Autodesk Fusion 360 part; units mm, degrees
(part 2 of 2)
sketch "Sketch5" plane through (0, 0, 0) normal (0, 0, 1) x (1, 0, 0)
  circle A0 centre (0, 0) radius 99.7546
  line L0 (-24.2133, 222.1165) -> (-40.213, 240.9922)
  arc A1 (-40.213, 240.9922) -> (-47.0298, 239.7551) centre (-43.2643, 238.4058) ccw
  line L1 (-47.0298, 239.7551) -> (-55.3768, 216.4612)
  arc A2 (-58.0942, 213.9503) -> (-55.3768, 216.4612) centre (-59.1424, 217.8105) ccw
  arc A3 (-58.0942, 213.9503) -> (-59.8641, 213.4618) centre (0, 0) ccw
  arc A4 (-63.4846, 214.2236) -> (-59.8641, 213.4618) centre (-60.9442, 217.3132) ccw
  line L2 (-63.4846, 214.2236) -> (-82.5975, 229.9391)
  arc A5 (-82.5975, 229.9391) -> (-89.084, 227.5047) centre (-85.138, 226.8494) ccw
  line L3 (-89.084, 227.5047) -> (-93.1375, 203.0946)
  arc A6 (-95.3629, 200.1389) -> (-93.1375, 203.0946) centre (-97.0835, 203.7499) ccw
  arc A7 (-95.3629, 200.1389) -> (-97.0171, 199.3423) centre (0, 0) ccw
  arc A8 (-100.7155, 199.4453) -> (-97.0171, 199.3423) centre (-98.7675, 202.9389) ccw
  line L4 (-100.7155, 199.4453) -> (-122.3274, 211.4955)
  arc A9 (-122.3274, 211.4955) -> (-128.2749, 207.942) centre (-124.2753, 208.0019) ccw
  line L5 (-128.2749, 207.942) -> (-127.9047, 183.2005)
  arc A10 (-129.5665, 179.8949) -> (-127.9047, 183.2005) centre (-131.9043, 183.1406) ccw
  arc A11 (-129.5665, 179.8949) -> (-131.0519, 178.8157) centre (0, 0) ccw
  arc A12 (-134.7093, 178.2567) -> (-131.0519, 178.8157) centre (-133.4164, 182.042) ccw
  line L6 (-134.7093, 178.2567) -> (-158.1255, 186.2543)
  arc A13 (-158.1255, 186.2543) -> (-163.3429, 181.6959) centre (-159.4183, 182.469) ccw
  line L7 (-163.3429, 181.6959) -> (-158.5609, 157.4181)
  arc A14 (-159.6058, 153.8689) -> (-158.5609, 157.4181) centre (-162.4855, 156.6451) ccw
  arc A15 (-159.6058, 153.8689) -> (-160.8746, 152.5418) centre (0, 0) ccw
  arc A16 (-164.3734, 151.3387) -> (-160.8746, 152.5418) centre (-163.7772, 155.2941) ccw
  line L8 (-164.3734, 151.3387) -> (-188.8413, 155.0267)
  arc A17 (-188.8413, 155.0267) -> (-193.161, 149.61) centre (-189.4375, 151.0714) ccw
  line L9 (-193.161, 149.61) -> (-184.1209, 126.5762)
  arc A18 (-184.5152, 122.8974) -> (-184.1209, 126.5762) centre (-187.8444, 125.1148) ccw
  arc A19 (-184.5152, 122.8974) -> (-185.5267, 121.3651) centre (0, 0) ccw
  arc A20 (-188.7544, 119.5567) -> (-185.5267, 121.3651) centre (-188.8741, 123.5549) ccw
  line L10 (-188.7544, 119.5567) -> (-213.4877, 118.8164)
  arc A21 (-213.4877, 118.8164) -> (-216.7707, 112.7155) centre (-213.368, 114.8182) ccw
  line L11 (-216.7707, 112.7155) -> (-203.763, 91.666)
  arc A22 (-203.4942, 87.9759) -> (-203.763, 91.666) centre (-207.1658, 89.5633) ccw
  arc A23 (-203.4942, 87.9759) -> (-204.2158, 86.2877) centre (0, 0) ccw
  arc A24 (-207.0687, 83.9319) -> (-204.2158, 86.2877) centre (-207.9004, 87.8445) ccw
  line L12 (-207.0687, 83.9319) -> (-231.2723, 78.7873)
  arc A25 (-231.2723, 78.7873) -> (-233.4133, 72.1982) centre (-230.4407, 74.8747) ccw
  line L13 (-233.4133, 72.1982) -> (-216.8561, 53.8096)
  arc A26 (-215.9327, 50.2268) -> (-216.8561, 53.8096) centre (-219.8287, 51.1331) ccw
  arc A27 (-215.9327, 50.2268) -> (-216.3412, 48.4369) centre (0, 0) ccw
  arc A28 (-218.7277, 45.6096) -> (-216.3412, 48.4369) centre (-220.2446, 49.3108) ccw
  line L14 (-218.7277, 45.6096) -> (-241.6237, 36.2259)
  arc A29 (-241.6237, 36.2259) -> (-242.5537, 29.3604) centre (-240.1068, 32.5247) ccw
  line L15 (-242.5537, 29.3604) -> (-222.9792, 14.2237)
  arc A30 (-221.4309, 10.8634) -> (-222.9792, 14.2237) centre (-225.4261, 11.0594) ccw
  arc A31 (-221.4309, 10.8634) -> (-221.5133, 9.0292) centre (0, 0) ccw
  arc A32 (-223.3565, 5.8213) -> (-221.5133, 9.0292) centre (-225.51, 9.1921) ccw
  line L16 (-223.3565, 5.8213) -> (-244.2091, -7.4998)
  arc A33 (-244.2091, -7.4998) -> (-243.8983, -14.4211) centre (-242.0557, -10.8707) ccw
  line L17 (-243.8983, -14.4211) -> (-221.9356, -25.8194)
  arc A34 (-219.8121, -28.8492) -> (-221.9356, -25.8194) centre (-223.7781, -29.3697) ccw
  arc A35 (-219.8121, -28.8492) -> (-219.5657, -30.6686) centre (0, 0) ccw
  arc A36 (-220.8065, -34.1541) -> (-219.5657, -30.6686) centre (-223.5272, -31.2219) ccw
  line L18 (-220.8065, -34.1541) -> (-238.9454, -50.9845)
  arc A37 (-238.9454, -50.9845) -> (-237.4037, -57.739) centre (-236.2247, -53.9167) ccw
  line L19 (-237.4037, -57.739) -> (-213.7587, -65.0326)
  arc A38 (-211.1285, -67.6345) -> (-213.7587, -65.0326) centre (-214.9378, -68.8548) ccw
  arc A39 (-211.1285, -67.6345) -> (-210.5611, -69.3807) centre (0, 0) ccw
  arc A40 (-211.1596, -73.0318) -> (-210.5611, -69.3807) centre (-214.3602, -70.6325) ccw
  line L20 (-211.1596, -73.0318) -> (-226.0018, -92.8305)
  arc A41 (-226.0018, -92.8305) -> (-223.2788, -99.2012) centre (-222.8013, -95.2298) ccw
  line L21 (-223.2788, -99.2012) -> (-198.7115, -102.1555)
  arc A42 (-195.6589, -104.2461) -> (-198.7115, -102.1555) centre (-199.1891, -106.1269) ccw
  arc A43 (-195.6589, -104.2461) -> (-194.7889, -105.8629) centre (0, 0) ccw
  arc A44 (-194.7259, -109.5622) -> (-194.7889, -105.8629) centre (-198.3034, -107.7729) ccw
  line L22 (-194.7259, -109.5622) -> (-205.7943, -131.6929)
  arc A45 (-205.7943, -131.6929) -> (-201.9776, -137.475) centre (-202.2168, -133.4822) ccw
  line L23 (-201.9776, -137.475) -> (-177.2776, -135.9952)
  arc A46 (-173.9007, -137.507) -> (-177.2776, -135.9952) centre (-177.0384, -139.988) ccw
  arc A47 (-173.9007, -137.507) -> (-172.756, -138.9425) centre (0, 0) ccw
  arc A48 (-172.0335, -142.5711) -> (-172.756, -138.9425) centre (-175.873, -141.4494) ccw
  line L24 (-172.0335, -142.5711) -> (-178.9725, -166.3225)
  arc A49 (-178.9725, -166.3225) -> (-174.1846, -171.3302) centre (-175.133, -167.4442) ccw
  line L25 (-174.1846, -171.3302) -> (-150.1458, -165.4638)
  arc A50 (-146.5533, -166.3484) -> (-150.1458, -165.4638) centre (-149.1975, -169.3498) ccw
  arc A51 (-146.5533, -166.3484) -> (-145.1706, -167.5564) centre (0, 0) ccw
  arc A52 (-143.8118, -170.9977) -> (-145.1706, -167.5564) centre (-147.7899, -170.5796) ccw
  line L26 (-143.8118, -170.9977) -> (-146.3983, -195.6064)
  arc A53 (-146.3983, -195.6064) -> (-140.7932, -199.6787) centre (-142.4202, -196.0245) ccw
  line L27 (-140.7932, -199.6787) -> (-118.1882, -189.6143)
  arc A54 (-114.4954, -189.8432) -> (-118.1882, -189.6143) centre (-116.5612, -193.2685) ccw
  arc A55 (-114.4954, -189.8432) -> (-112.9193, -190.7849) centre (0, 0) ccw
  arc A56 (-110.9678, -193.9283) -> (-112.9193, -190.7849) centre (-114.9567, -194.2272) ccw
  line L28 (-110.9678, -193.9283) -> (-109.1187, -218.6034)
  arc A57 (-109.1187, -218.6034) -> (-102.8766, -221.6094) centre (-105.1299, -218.3045) ccw
  line L29 (-102.8766, -221.6094) -> (-82.4319, -207.6704)
  arc A58 (-78.7576, -207.2363) -> (-82.4319, -207.6704) centre (-80.1786, -210.9754) ccw
  arc A59 (-78.7576, -207.2363) -> (-77.0387, -207.8815) centre (0, 0) ccw
  arc A60 (-74.5573, -210.6258) -> (-77.0387, -207.8815) centre (-78.4287, -211.6322) ccw
  line L30 (-74.5573, -210.6258) -> (-68.332, -234.5742)
  arc A61 (-68.332, -234.5742) -> (-61.6534, -236.4174) centre (-64.4606, -233.5679) ccw
  line L31 (-61.6534, -236.4174) -> (-44.0262, -219.0519)
  arc A62 (-40.4885, -217.9687) -> (-44.0262, -219.0519) centre (-41.219, -221.9014) ccw
  arc A63 (-40.4885, -217.9687) -> (-38.682, -218.2965) centre (0, 0) ccw
  arc A64 (-35.7505, -220.5537) -> (-38.682, -218.2965) centre (-39.3799, -222.2351) ccw
  line L32 (-35.7505, -220.5537) -> (-25.349, -243.0057)
  arc A65 (-25.349, -243.0057) -> (-18.4487, -243.6267) centre (-21.7196, -241.3242) ccw
  line L33 (-18.4487, -243.6267) -> (-4.2055, -223.3928)
  arc A66 (-0.918, -221.6953) -> (-4.2055, -223.3928) centre (-0.9346, -225.6953) ccw
  arc A67 (-0.918, -221.6953) -> (0.918, -221.6953) centre (0, 0) ccw
  arc A68 (4.2055, -223.3928) -> (0.918, -221.6953) centre (0.9346, -225.6953) ccw
  line L34 (4.2055, -223.3928) -> (18.4487, -243.6267)
  arc A69 (18.4487, -243.6267) -> (25.349, -243.0057) centre (21.7196, -241.3242) ccw
  line L35 (25.349, -243.0057) -> (35.7505, -220.5537)
  arc A70 (38.682, -218.2965) -> (35.7505, -220.5537) centre (39.3799, -222.2351) ccw
  arc A71 (38.682, -218.2965) -> (40.4885, -217.9687) centre (0, 0) ccw
  arc A72 (44.0262, -219.0519) -> (40.4885, -217.9687) centre (41.219, -221.9014) ccw
  line L36 (44.0262, -219.0519) -> (61.6534, -236.4174)
  arc A73 (61.6534, -236.4174) -> (68.332, -234.5742) centre (64.4606, -233.5679) ccw
  line L37 (68.332, -234.5742) -> (74.5573, -210.6258)
  arc A74 (77.0387, -207.8815) -> (74.5573, -210.6258) centre (78.4287, -211.6322) ccw
  arc A75 (77.0387, -207.8815) -> (78.7576, -207.2363) centre (0, 0) ccw
  arc A76 (82.4319, -207.6704) -> (78.7576, -207.2363) centre (80.1786, -210.9754) ccw
  line L38 (82.4319, -207.6704) -> (102.8766, -221.6094)
  arc A77 (102.8766, -221.6094) -> (109.1187, -218.6034) centre (105.1299, -218.3045) ccw
  line L39 (109.1187, -218.6034) -> (110.9678, -193.9283)
  arc A78 (112.9193, -190.7849) -> (110.9678, -193.9283) centre (114.9567, -194.2272) ccw
  arc A79 (112.9193, -190.7849) -> (114.4954, -189.8432) centre (0, 0) ccw
  arc A80 (118.1882, -189.6143) -> (114.4954, -189.8432) centre (116.5612, -193.2685) ccw
  line L40 (118.1882, -189.6143) -> (140.7932, -199.6787)
  arc A81 (140.7932, -199.6787) -> (146.3983, -195.6064) centre (142.4202, -196.0245) ccw
  line L41 (146.3983, -195.6064) -> (143.8118, -170.9977)
  arc A82 (145.1706, -167.5564) -> (143.8118, -170.9977) centre (147.7899, -170.5796) ccw
  arc A83 (145.1706, -167.5564) -> (146.5533, -166.3484) centre (0, 0) ccw
  arc A84 (150.1458, -165.4638) -> (146.5533, -166.3484) centre (149.1975, -169.3498) ccw
  line L42 (150.1458, -165.4638) -> (174.1846, -171.3302)
  arc A85 (174.1846, -171.3302) -> (178.9725, -166.3225) centre (175.133, -167.4442) ccw
  line L43 (178.9725, -166.3225) -> (172.0335, -142.5711)
  arc A86 (172.756, -138.9425) -> (172.0335, -142.5711) centre (175.873, -141.4494) ccw
  arc A87 (172.756, -138.9425) -> (173.9007, -137.507) centre (0, 0) ccw
  arc A88 (177.2776, -135.9952) -> (173.9007, -137.507) centre (177.0384, -139.988) ccw
  line L44 (177.2776, -135.9952) -> (201.9776, -137.475)
  arc A89 (201.9776, -137.475) -> (205.7943, -131.6929) centre (202.2168, -133.4822) ccw
  line L45 (205.7943, -131.6929) -> (194.7259, -109.5622)
  arc A90 (194.7889, -105.8629) -> (194.7259, -109.5622) centre (198.3034, -107.7729) ccw
  arc A91 (194.7889, -105.8629) -> (195.6589, -104.2461) centre (0, 0) ccw
  arc A92 (198.7115, -102.1555) -> (195.6589, -104.2461) centre (199.1891, -106.1269) ccw
  line L46 (198.7115, -102.1555) -> (223.2788, -99.2012)
  arc A93 (223.2788, -99.2012) -> (226.0018, -92.8305) centre (222.8013, -95.2298) ccw
  line L47 (226.0018, -92.8305) -> (211.1596, -73.0318)
  arc A94 (210.5611, -69.3807) -> (211.1596, -73.0318) centre (214.3602, -70.6325) ccw
  arc A95 (210.5611, -69.3807) -> (211.1285, -67.6345) centre (0, 0) ccw
  arc A96 (213.7587, -65.0326) -> (211.1285, -67.6345) centre (214.9378, -68.8548) ccw
  line L48 (213.7587, -65.0326) -> (237.4037, -57.739)
  arc A97 (237.4037, -57.739) -> (238.9454, -50.9845) centre (236.2247, -53.9167) ccw
  line L49 (238.9454, -50.9845) -> (220.8065, -34.1541)
  arc A98 (219.5657, -30.6686) -> (220.8065, -34.1541) centre (223.5272, -31.2219) ccw
  arc A99 (219.5657, -30.6686) -> (219.8121, -28.8492) centre (0, 0) ccw
  arc A100 (221.9356, -25.8194) -> (219.8121, -28.8492) centre (223.7781, -29.3697) ccw
  line L50 (221.9356, -25.8194) -> (243.8983, -14.4211)
  arc A101 (243.8983, -14.4211) -> (244.2091, -7.4998) centre (242.0557, -10.8707) ccw
  line L51 (244.2091, -7.4998) -> (223.3565, 5.8213)
  arc A102 (221.5133, 9.0292) -> (223.3565, 5.8213) centre (225.51, 9.1921) ccw
  arc A103 (221.5133, 9.0292) -> (221.4309, 10.8634) centre (0, 0) ccw
  arc A104 (222.9792, 14.2237) -> (221.4309, 10.8634) centre (225.4261, 11.0594) ccw
  line L52 (222.9792, 14.2237) -> (242.5537, 29.3604)
  arc A105 (242.5537, 29.3604) -> (241.6237, 36.2259) centre (240.1068, 32.5247) ccw
  line L53 (241.6237, 36.2259) -> (218.7277, 45.6096)
  arc A106 (216.3412, 48.4369) -> (218.7277, 45.6096) centre (220.2446, 49.3108) ccw
  arc A107 (216.3412, 48.4369) -> (215.9327, 50.2268) centre (0, 0) ccw
  arc A108 (216.8561, 53.8096) -> (215.9327, 50.2268) centre (219.8287, 51.1331) ccw
  line L54 (216.8561, 53.8096) -> (233.4133, 72.1982)
  arc A109 (233.4133, 72.1982) -> (231.2723, 78.7873) centre (230.4407, 74.8747) ccw
  line L55 (231.2723, 78.7873) -> (207.0687, 83.9319)
  arc A110 (204.2158, 86.2877) -> (207.0687, 83.9319) centre (207.9004, 87.8445) ccw
  arc A111 (204.2158, 86.2877) -> (203.4942, 87.9759) centre (0, 0) ccw
  arc A112 (203.763, 91.666) -> (203.4942, 87.9759) centre (207.1658, 89.5633) ccw
  line L56 (203.763, 91.666) -> (216.7707, 112.7155)
  arc A113 (216.7707, 112.7155) -> (213.4877, 118.8164) centre (213.368, 114.8182) ccw
  line L57 (213.4877, 118.8164) -> (188.7544, 119.5567)
  arc A114 (185.5267, 121.3651) -> (188.7544, 119.5567) centre (188.8741, 123.5549) ccw
  arc A115 (185.5267, 121.3651) -> (184.5152, 122.8974) centre (0, 0) ccw
  arc A116 (184.1209, 126.5762) -> (184.5152, 122.8974) centre (187.8444, 125.1148) ccw
  line L58 (184.1209, 126.5762) -> (193.161, 149.61)
  arc A117 (193.161, 149.61) -> (188.8413, 155.0267) centre (189.4375, 151.0714) ccw
  line L59 (188.8413, 155.0267) -> (164.3734, 151.3387)
  arc A118 (160.8746, 152.5418) -> (164.3734, 151.3387) centre (163.7772, 155.2941) ccw
  arc A119 (160.8746, 152.5418) -> (159.6058, 153.8689) centre (0, 0) ccw
  arc A120 (158.5609, 157.4181) -> (159.6058, 153.8689) centre (162.4855, 156.6451) ccw
  line L60 (158.5609, 157.4181) -> (163.3429, 181.6959)
  arc A121 (163.3429, 181.6959) -> (158.1255, 186.2543) centre (159.4183, 182.469) ccw
  line L61 (158.1255, 186.2543) -> (134.7093, 178.2567)
  arc A122 (131.0519, 178.8157) -> (134.7093, 178.2567) centre (133.4164, 182.042) ccw
  arc A123 (131.0519, 178.8157) -> (129.5665, 179.8949) centre (0, 0) ccw
  arc A124 (127.9047, 183.2005) -> (129.5665, 179.8949) centre (131.9043, 183.1406) ccw
  line L62 (127.9047, 183.2005) -> (128.2749, 207.942)
  arc A125 (128.2749, 207.942) -> (122.3274, 211.4955) centre (124.2753, 208.0019) ccw
  line L63 (122.3274, 211.4955) -> (100.7155, 199.4453)
  arc A126 (97.0171, 199.3423) -> (100.7155, 199.4453) centre (98.7675, 202.9389) ccw
  arc A127 (97.0171, 199.3423) -> (95.3629, 200.1389) centre (0, 0) ccw
  arc A128 (93.1375, 203.0946) -> (95.3629, 200.1389) centre (97.0835, 203.7499) ccw
  line L64 (93.1375, 203.0946) -> (89.084, 227.5047)
  arc A129 (89.084, 227.5047) -> (82.5975, 229.9391) centre (85.138, 226.8494) ccw
  line L65 (82.5975, 229.9391) -> (63.4846, 214.2236)
  arc A130 (59.8641, 213.4618) -> (63.4846, 214.2236) centre (60.9442, 217.3132) ccw
  arc A131 (59.8641, 213.4618) -> (58.0942, 213.9503) centre (0, 0) ccw
  arc A132 (55.3768, 216.4612) -> (58.0942, 213.9503) centre (59.1424, 217.8105) ccw
  line L66 (55.3768, 216.4612) -> (47.0298, 239.7551)
  arc A133 (47.0298, 239.7551) -> (40.213, 240.9922) centre (43.2643, 238.4058) ccw
  line L67 (40.213, 240.9922) -> (24.2133, 222.1165)
  arc A134 (20.7869, 220.7205) -> (24.2133, 222.1165) centre (21.162, 224.7029) ccw
  arc A135 (20.7869, 220.7205) -> (18.9583, 220.8851) centre (0, 0) ccw
  arc A136 (15.8363, 222.8705) -> (18.9583, 220.8851) centre (19.3004, 224.8705) ccw
  line L68 (15.8363, 222.8705) -> (3.4641, 244.2997)
  arc A137 (3.4641, 244.2997) -> (-3.4641, 244.2997) centre (0, 242.2997) ccw
  line L69 (-3.4641, 244.2997) -> (-15.8363, 222.8705)
  arc A138 (-18.9583, 220.8851) -> (-15.8363, 222.8705) centre (-19.3004, 224.8705) ccw
  arc A139 (-18.9583, 220.8851) -> (-20.7869, 220.7205) centre (0, 0) ccw
  arc A140 (-24.2133, 222.1165) -> (-20.7869, 220.7205) centre (-21.162, 224.7029) ccw
  circle A141 centre (0, 0) radius 274.7781
  constraint coincident A0.centre A3.centre
extrude "Extrude5" add sketch "Sketch5" along normal blind 50 contours L0 A1 L1 A2 A3 A4 L2 A5 L3 A6 A7 A8 L4 A9 L5 A10 A11 A12 L6 A13 L7 A14 A15 A16 L8 A17 L9 A18 A19 A20 L10 A21 L11 A22 A23 A24 L12 A25 L13 A26 A27 A28 L14 A29 L15 A30 A31 A32 L16 A33 L17 A34 A35 A36 L18 A37 L19 A38 A39 A40 L20 A41 L21 A42 A43 A44 L22 A45 L23 A46 A47 A48 L24 A49 L25 A50 A51 A52 L26 A53 L27 A54 A55 A56 L28 A57 L29 A58 A59 A60 L30 A61 L31 A62 A63 A64 L32 A65 L33 A66 A67 A68 L34 A69 L35 A70 A71 A72 L36 A73 L37 A74 A75 A76 L38 A77 L39 A78 A79 A80 L40 A81 L41 A82 A83 A84 L42 A85 L43 A86 A87 A88 L44 A89 L45 A90 A91 A92 L46 A93 L47 A94 A95 A96 L48 A97 L49 A98 A99 A100 L50 A101 L51 A102 A103 A104 L52 A105 L53 A106 A107 A108 L54 A109 L55 A110 A111 A112 L56 A113 L57 A114 A115 A116 L58 A117 L59 A118 A119 A120 L60 A121 L61 A122 A123 A124 L62 A125 L63 A126 A127 A128 L64 A129 L65 A130 A131 A132 L66 A133 L67 A134 A135 A136 L68 A137 L69 A138 A139 A140 | A141 bodies 1
sketch "Sketch6" plane through (0, 0, -1200) normal (0, 0, -1) x (-1, 0, 0)
  circle A0 centre (0, 0) radius 100.098
  line L0 (55.3768, 216.4612) -> (47.0298, 239.7551)
  arc A1 (47.0298, 239.7551) -> (40.213, 240.9922) centre (43.2643, 238.4058) ccw
  line L1 (40.213, 240.9922) -> (24.2133, 222.1165)
  arc A2 (20.7869, 220.7205) -> (24.2133, 222.1165) centre (21.162, 224.7029) ccw
  arc A3 (20.7869, 220.7205) -> (18.9583, 220.8851) centre (0, 0) ccw
  arc A4 (15.8363, 222.8705) -> (18.9583, 220.8851) centre (19.3004, 224.8705) ccw
  line L2 (15.8363, 222.8705) -> (3.4641, 244.2997)
  arc A5 (3.4641, 244.2997) -> (-3.4641, 244.2997) centre (0, 242.2997) ccw
  line L3 (-3.4641, 244.2997) -> (-15.8363, 222.8705)
  arc A6 (-18.9583, 220.8851) -> (-15.8363, 222.8705) centre (-19.3004, 224.8705) ccw
  arc A7 (-18.9583, 220.8851) -> (-20.7869, 220.7205) centre (0, 0) ccw
  arc A8 (-24.2133, 222.1165) -> (-20.7869, 220.7205) centre (-21.162, 224.7029) ccw
  line L4 (-24.2133, 222.1165) -> (-40.213, 240.9922)
  arc A9 (-40.213, 240.9922) -> (-47.0298, 239.7551) centre (-43.2643, 238.4058) ccw
  line L5 (-47.0298, 239.7551) -> (-55.3768, 216.4612)
  arc A10 (-58.0942, 213.9503) -> (-55.3768, 216.4612) centre (-59.1424, 217.8105) ccw
  arc A11 (-58.0942, 213.9503) -> (-59.8641, 213.4618) centre (0, 0) ccw
  arc A12 (-63.4846, 214.2236) -> (-59.8641, 213.4618) centre (-60.9442, 217.3132) ccw
  line L6 (-63.4846, 214.2236) -> (-82.5975, 229.9391)
  arc A13 (-82.5975, 229.9391) -> (-89.084, 227.5047) centre (-85.138, 226.8494) ccw
  line L7 (-89.084, 227.5047) -> (-93.1375, 203.0946)
  arc A14 (-95.3629, 200.1389) -> (-93.1375, 203.0946) centre (-97.0835, 203.7499) ccw
  arc A15 (-95.3629, 200.1389) -> (-97.0171, 199.3423) centre (0, 0) ccw
  arc A16 (-100.7155, 199.4453) -> (-97.0171, 199.3423) centre (-98.7675, 202.9389) ccw
  line L8 (-100.7155, 199.4453) -> (-122.3274, 211.4955)
  arc A17 (-122.3274, 211.4955) -> (-128.2749, 207.942) centre (-124.2753, 208.0019) ccw
  line L9 (-128.2749, 207.942) -> (-127.9047, 183.2005)
  arc A18 (-129.5665, 179.8949) -> (-127.9047, 183.2005) centre (-131.9043, 183.1406) ccw
  arc A19 (-129.5665, 179.8949) -> (-131.0519, 178.8157) centre (0, 0) ccw
  arc A20 (-134.7093, 178.2567) -> (-131.0519, 178.8157) centre (-133.4164, 182.042) ccw
  line L10 (-134.7093, 178.2567) -> (-158.1255, 186.2543)
  arc A21 (-158.1255, 186.2543) -> (-163.3429, 181.6959) centre (-159.4183, 182.469) ccw
  line L11 (-163.3429, 181.6959) -> (-158.5609, 157.4181)
  arc A22 (-159.6058, 153.8689) -> (-158.5609, 157.4181) centre (-162.4855, 156.6451) ccw
  arc A23 (-159.6058, 153.8689) -> (-160.8746, 152.5418) centre (0, 0) ccw
  arc A24 (-164.3734, 151.3387) -> (-160.8746, 152.5418) centre (-163.7772, 155.2941) ccw
  line L12 (-164.3734, 151.3387) -> (-188.8413, 155.0267)
  arc A25 (-188.8413, 155.0267) -> (-193.161, 149.61) centre (-189.4375, 151.0714) ccw
  line L13 (-193.161, 149.61) -> (-184.1209, 126.5762)
  arc A26 (-184.5152, 122.8974) -> (-184.1209, 126.5762) centre (-187.8444, 125.1148) ccw
  arc A27 (-184.5152, 122.8974) -> (-185.5267, 121.3651) centre (0, 0) ccw
  arc A28 (-188.7544, 119.5567) -> (-185.5267, 121.3651) centre (-188.8741, 123.5549) ccw
  line L14 (-188.7544, 119.5567) -> (-213.4877, 118.8164)
  arc A29 (-213.4877, 118.8164) -> (-216.7707, 112.7155) centre (-213.368, 114.8182) ccw
  line L15 (-216.7707, 112.7155) -> (-203.763, 91.666)
  arc A30 (-203.4942, 87.9759) -> (-203.763, 91.666) centre (-207.1658, 89.5633) ccw
  arc A31 (-203.4942, 87.9759) -> (-204.2158, 86.2877) centre (0, 0) ccw
  arc A32 (-207.0687, 83.9319) -> (-204.2158, 86.2877) centre (-207.9004, 87.8445) ccw
  line L16 (-207.0687, 83.9319) -> (-231.2723, 78.7873)
  arc A33 (-231.2723, 78.7873) -> (-233.4133, 72.1982) centre (-230.4407, 74.8747) ccw
  line L17 (-233.4133, 72.1982) -> (-216.8561, 53.8096)
  arc A34 (-215.9327, 50.2268) -> (-216.8561, 53.8096) centre (-219.8287, 51.1331) ccw
  arc A35 (-215.9327, 50.2268) -> (-216.3412, 48.4369) centre (0, 0) ccw
  arc A36 (-218.7277, 45.6096) -> (-216.3412, 48.4369) centre (-220.2446, 49.3108) ccw
  line L18 (-218.7277, 45.6096) -> (-241.6237, 36.2259)
  arc A37 (-241.6237, 36.2259) -> (-242.5537, 29.3604) centre (-240.1068, 32.5247) ccw
  line L19 (-242.5537, 29.3604) -> (-222.9792, 14.2237)
  arc A38 (-221.4309, 10.8634) -> (-222.9792, 14.2237) centre (-225.4261, 11.0594) ccw
  arc A39 (-221.4309, 10.8634) -> (-221.5133, 9.0292) centre (0, 0) ccw
  arc A40 (-223.3565, 5.8213) -> (-221.5133, 9.0292) centre (-225.51, 9.1921) ccw
  line L20 (-223.3565, 5.8213) -> (-244.2091, -7.4998)
  arc A41 (-244.2091, -7.4998) -> (-243.8983, -14.4211) centre (-242.0557, -10.8707) ccw
  line L21 (-243.8983, -14.4211) -> (-221.9356, -25.8194)
  arc A42 (-219.8121, -28.8492) -> (-221.9356, -25.8194) centre (-223.7781, -29.3697) ccw
  arc A43 (-219.8121, -28.8492) -> (-219.5657, -30.6686) centre (0, 0) ccw
  arc A44 (-220.8065, -34.1541) -> (-219.5657, -30.6686) centre (-223.5272, -31.2219) ccw
  line L22 (-220.8065, -34.1541) -> (-238.9454, -50.9845)
  arc A45 (-238.9454, -50.9845) -> (-237.4037, -57.739) centre (-236.2247, -53.9167) ccw
  line L23 (-237.4037, -57.739) -> (-213.7587, -65.0326)
  arc A46 (-211.1285, -67.6345) -> (-213.7587, -65.0326) centre (-214.9378, -68.8548) ccw
  arc A47 (-211.1285, -67.6345) -> (-210.5611, -69.3807) centre (0, 0) ccw
  arc A48 (-211.1596, -73.0318) -> (-210.5611, -69.3807) centre (-214.3602, -70.6325) ccw
  line L24 (-211.1596, -73.0318) -> (-226.0018, -92.8305)
  arc A49 (-226.0018, -92.8305) -> (-223.2788, -99.2012) centre (-222.8013, -95.2298) ccw
  line L25 (-223.2788, -99.2012) -> (-198.7115, -102.1555)
  arc A50 (-195.6589, -104.2461) -> (-198.7115, -102.1555) centre (-199.1891, -106.1269) ccw
  arc A51 (-195.6589, -104.2461) -> (-194.7889, -105.8629) centre (0, 0) ccw
  arc A52 (-194.7259, -109.5622) -> (-194.7889, -105.8629) centre (-198.3034, -107.7729) ccw
  line L26 (-194.7259, -109.5622) -> (-205.7943, -131.6929)
  arc A53 (-205.7943, -131.6929) -> (-201.9776, -137.475) centre (-202.2168, -133.4822) ccw
  line L27 (-201.9776, -137.475) -> (-177.2776, -135.9952)
  arc A54 (-173.9007, -137.507) -> (-177.2776, -135.9952) centre (-177.0384, -139.988) ccw
  arc A55 (-173.9007, -137.507) -> (-172.756, -138.9425) centre (0, 0) ccw
  arc A56 (-172.0335, -142.5711) -> (-172.756, -138.9425) centre (-175.873, -141.4494) ccw
  line L28 (-172.0335, -142.5711) -> (-178.9725, -166.3225)
  arc A57 (-178.9725, -166.3225) -> (-174.1846, -171.3302) centre (-175.133, -167.4442) ccw
  line L29 (-174.1846, -171.3302) -> (-150.1458, -165.4638)
  arc A58 (-146.5533, -166.3484) -> (-150.1458, -165.4638) centre (-149.1975, -169.3498) ccw
  arc A59 (-146.5533, -166.3484) -> (-145.1706, -167.5564) centre (0, 0) ccw
  arc A60 (-143.8118, -170.9977) -> (-145.1706, -167.5564) centre (-147.7899, -170.5796) ccw
  line L30 (-143.8118, -170.9977) -> (-146.3983, -195.6064)
  arc A61 (-146.3983, -195.6064) -> (-140.7932, -199.6787) centre (-142.4202, -196.0245) ccw
  line L31 (-140.7932, -199.6787) -> (-118.1882, -189.6143)
  arc A62 (-114.4954, -189.8432) -> (-118.1882, -189.6143) centre (-116.5612, -193.2685) ccw
  arc A63 (-114.4954, -189.8432) -> (-112.9193, -190.7849) centre (0, 0) ccw
  arc A64 (-110.9678, -193.9283) -> (-112.9193, -190.7849) centre (-114.9567, -194.2272) ccw
  line L32 (-110.9678, -193.9283) -> (-109.1187, -218.6034)
  arc A65 (-109.1187, -218.6034) -> (-102.8766, -221.6094) centre (-105.1299, -218.3045) ccw
  line L33 (-102.8766, -221.6094) -> (-82.4319, -207.6704)
  arc A66 (-78.7576, -207.2363) -> (-82.4319, -207.6704) centre (-80.1786, -210.9754) ccw
  arc A67 (-78.7576, -207.2363) -> (-77.0387, -207.8815) centre (0, 0) ccw
  arc A68 (-74.5573, -210.6258) -> (-77.0387, -207.8815) centre (-78.4287, -211.6322) ccw
  line L34 (-74.5573, -210.6258) -> (-68.332, -234.5742)
  arc A69 (-68.332, -234.5742) -> (-61.6534, -236.4174) centre (-64.4606, -233.5679) ccw
  line L35 (-61.6534, -236.4174) -> (-44.0262, -219.0519)
  arc A70 (-40.4885, -217.9687) -> (-44.0262, -219.0519) centre (-41.219, -221.9014) ccw
  arc A71 (-40.4885, -217.9687) -> (-38.682, -218.2965) centre (0, 0) ccw
  arc A72 (-35.7505, -220.5537) -> (-38.682, -218.2965) centre (-39.3799, -222.2351) ccw
  line L36 (-35.7505, -220.5537) -> (-25.349, -243.0057)
  arc A73 (-25.349, -243.0057) -> (-18.4487, -243.6267) centre (-21.7196, -241.3242) ccw
  line L37 (-18.4487, -243.6267) -> (-4.2055, -223.3928)
  arc A74 (-0.918, -221.6953) -> (-4.2055, -223.3928) centre (-0.9346, -225.6953) ccw
  arc A75 (-0.918, -221.6953) -> (0.918, -221.6953) centre (0, 0) ccw
  arc A76 (4.2055, -223.3928) -> (0.918, -221.6953) centre (0.9346, -225.6953) ccw
  line L38 (4.2055, -223.3928) -> (18.4487, -243.6267)
  arc A77 (18.4487, -243.6267) -> (25.349, -243.0057) centre (21.7196, -241.3242) ccw
  line L39 (25.349, -243.0057) -> (35.7505, -220.5537)
  arc A78 (38.682, -218.2965) -> (35.7505, -220.5537) centre (39.3799, -222.2351) ccw
  arc A79 (38.682, -218.2965) -> (40.4885, -217.9687) centre (0, 0) ccw
  arc A80 (44.0262, -219.0519) -> (40.4885, -217.9687) centre (41.219, -221.9014) ccw
  line L40 (44.0262, -219.0519) -> (61.6534, -236.4174)
  arc A81 (61.6534, -236.4174) -> (68.332, -234.5742) centre (64.4606, -233.5679) ccw
  line L41 (68.332, -234.5742) -> (74.5573, -210.6258)
  arc A82 (77.0387, -207.8815) -> (74.5573, -210.6258) centre (78.4287, -211.6322) ccw
  arc A83 (77.0387, -207.8815) -> (78.7576, -207.2363) centre (0, 0) ccw
  arc A84 (82.4319, -207.6704) -> (78.7576, -207.2363) centre (80.1786, -210.9754) ccw
  line L42 (82.4319, -207.6704) -> (102.8766, -221.6094)
  arc A85 (102.8766, -221.6094) -> (109.1187, -218.6034) centre (105.1299, -218.3045) ccw
  line L43 (109.1187, -218.6034) -> (110.9678, -193.9283)
  arc A86 (112.9193, -190.7849) -> (110.9678, -193.9283) centre (114.9567, -194.2272) ccw
  arc A87 (112.9193, -190.7849) -> (114.4954, -189.8432) centre (0, 0) ccw
  arc A88 (118.1882, -189.6143) -> (114.4954, -189.8432) centre (116.5612, -193.2685) ccw
  line L44 (118.1882, -189.6143) -> (140.7932, -199.6787)
  arc A89 (140.7932, -199.6787) -> (146.3983, -195.6064) centre (142.4202, -196.0245) ccw
  line L45 (146.3983, -195.6064) -> (143.8118, -170.9977)
  arc A90 (145.1706, -167.5564) -> (143.8118, -170.9977) centre (147.7899, -170.5796) ccw
  arc A91 (145.1706, -167.5564) -> (146.5533, -166.3484) centre (0, 0) ccw
  arc A92 (150.1458, -165.4638) -> (146.5533, -166.3484) centre (149.1975, -169.3498) ccw
  line L46 (150.1458, -165.4638) -> (174.1846, -171.3302)
  arc A93 (174.1846, -171.3302) -> (178.9725, -166.3225) centre (175.133, -167.4442) ccw
  line L47 (178.9725, -166.3225) -> (172.0335, -142.5711)
  arc A94 (172.756, -138.9425) -> (172.0335, -142.5711) centre (175.873, -141.4494) ccw
  arc A95 (172.756, -138.9425) -> (173.9007, -137.507) centre (0, 0) ccw
  arc A96 (177.2776, -135.9952) -> (173.9007, -137.507) centre (177.0384, -139.988) ccw
  line L48 (177.2776, -135.9952) -> (201.9776, -137.475)
  arc A97 (201.9776, -137.475) -> (205.7943, -131.6929) centre (202.2168, -133.4822) ccw
  line L49 (205.7943, -131.6929) -> (194.7259, -109.5622)
  arc A98 (194.7889, -105.8629) -> (194.7259, -109.5622) centre (198.3034, -107.7729) ccw
  arc A99 (194.7889, -105.8629) -> (195.6589, -104.2461) centre (0, 0) ccw
  arc A100 (198.7115, -102.1555) -> (195.6589, -104.2461) centre (199.1891, -106.1269) ccw
  line L50 (198.7115, -102.1555) -> (223.2788, -99.2012)
  arc A101 (223.2788, -99.2012) -> (226.0018, -92.8305) centre (222.8013, -95.2298) ccw
  line L51 (226.0018, -92.8305) -> (211.1596, -73.0318)
  arc A102 (210.5611, -69.3807) -> (211.1596, -73.0318) centre (214.3602, -70.6325) ccw
  arc A103 (210.5611, -69.3807) -> (211.1285, -67.6345) centre (0, 0) ccw
  arc A104 (213.7587, -65.0326) -> (211.1285, -67.6345) centre (214.9378, -68.8548) ccw
  line L52 (213.7587, -65.0326) -> (237.4037, -57.739)
  arc A105 (237.4037, -57.739) -> (238.9454, -50.9845) centre (236.2247, -53.9167) ccw
  line L53 (238.9454, -50.9845) -> (220.8065, -34.1541)
  arc A106 (219.5657, -30.6686) -> (220.8065, -34.1541) centre (223.5272, -31.2219) ccw
  arc A107 (219.5657, -30.6686) -> (219.8121, -28.8492) centre (0, 0) ccw
  arc A108 (221.9356, -25.8194) -> (219.8121, -28.8492) centre (223.7781, -29.3697) ccw
  line L54 (221.9356, -25.8194) -> (243.8983, -14.4211)
  arc A109 (243.8983, -14.4211) -> (244.2091, -7.4998) centre (242.0557, -10.8707) ccw
  line L55 (244.2091, -7.4998) -> (223.3565, 5.8213)
  arc A110 (221.5133, 9.0292) -> (223.3565, 5.8213) centre (225.51, 9.1921) ccw
  arc A111 (221.5133, 9.0292) -> (221.4309, 10.8634) centre (0, 0) ccw
  arc A112 (222.9792, 14.2237) -> (221.4309, 10.8634) centre (225.4261, 11.0594) ccw
  line L56 (222.9792, 14.2237) -> (242.5537, 29.3604)
  arc A113 (242.5537, 29.3604) -> (241.6237, 36.2259) centre (240.1068, 32.5247) ccw
  line L57 (241.6237, 36.2259) -> (218.7277, 45.6096)
  arc A114 (216.3412, 48.4369) -> (218.7277, 45.6096) centre (220.2446, 49.3108) ccw
  arc A115 (216.3412, 48.4369) -> (215.9327, 50.2268) centre (0, 0) ccw
  arc A116 (216.8561, 53.8096) -> (215.9327, 50.2268) centre (219.8287, 51.1331) ccw
  line L58 (216.8561, 53.8096) -> (233.4133, 72.1982)
  arc A117 (233.4133, 72.1982) -> (231.2723, 78.7873) centre (230.4407, 74.8747) ccw
  line L59 (231.2723, 78.7873) -> (207.0687, 83.9319)
  arc A118 (204.2158, 86.2877) -> (207.0687, 83.9319) centre (207.9004, 87.8445) ccw
  arc A119 (204.2158, 86.2877) -> (203.4942, 87.9759) centre (0, 0) ccw
  arc A120 (203.763, 91.666) -> (203.4942, 87.9759) centre (207.1658, 89.5633) ccw
  line L60 (203.763, 91.666) -> (216.7707, 112.7155)
  arc A121 (216.7707, 112.7155) -> (213.4877, 118.8164) centre (213.368, 114.8182) ccw
  line L61 (213.4877, 118.8164) -> (188.7544, 119.5567)
  arc A122 (185.5267, 121.3651) -> (188.7544, 119.5567) centre (188.8741, 123.5549) ccw
  arc A123 (185.5267, 121.3651) -> (184.5152, 122.8974) centre (0, 0) ccw
  arc A124 (184.1209, 126.5762) -> (184.5152, 122.8974) centre (187.8444, 125.1148) ccw
  line L62 (184.1209, 126.5762) -> (193.161, 149.61)
  arc A125 (193.161, 149.61) -> (188.8413, 155.0267) centre (189.4375, 151.0714) ccw
  line L63 (188.8413, 155.0267) -> (164.3734, 151.3387)
  arc A126 (160.8746, 152.5418) -> (164.3734, 151.3387) centre (163.7772, 155.2941) ccw
  arc A127 (160.8746, 152.5418) -> (159.6058, 153.8689) centre (0, 0) ccw
  arc A128 (158.5609, 157.4181) -> (159.6058, 153.8689) centre (162.4855, 156.6451) ccw
  line L64 (158.5609, 157.4181) -> (163.3429, 181.6959)
  arc A129 (163.3429, 181.6959) -> (158.1255, 186.2543) centre (159.4183, 182.469) ccw
  line L65 (158.1255, 186.2543) -> (134.7093, 178.2567)
  arc A130 (131.0519, 178.8157) -> (134.7093, 178.2567) centre (133.4164, 182.042) ccw
  arc A131 (131.0519, 178.8157) -> (129.5665, 179.8949) centre (0, 0) ccw
  arc A132 (127.9047, 183.2005) -> (129.5665, 179.8949) centre (131.9043, 183.1406) ccw
  line L66 (127.9047, 183.2005) -> (128.2749, 207.942)
  arc A133 (128.2749, 207.942) -> (122.3274, 211.4955) centre (124.2753, 208.0019) ccw
  line L67 (122.3274, 211.4955) -> (100.7155, 199.4453)
  arc A134 (97.0171, 199.3423) -> (100.7155, 199.4453) centre (98.7675, 202.9389) ccw
  arc A135 (97.0171, 199.3423) -> (95.3629, 200.1389) centre (0, 0) ccw
  arc A136 (93.1375, 203.0946) -> (95.3629, 200.1389) centre (97.0835, 203.7499) ccw
  line L68 (93.1375, 203.0946) -> (89.084, 227.5047)
  arc A137 (89.084, 227.5047) -> (82.5975, 229.9391) centre (85.138, 226.8494) ccw
  line L69 (82.5975, 229.9391) -> (63.4846, 214.2236)
  arc A138 (59.8641, 213.4618) -> (63.4846, 214.2236) centre (60.9442, 217.3132) ccw
  arc A139 (59.8641, 213.4618) -> (58.0942, 213.9503) centre (0, 0) ccw
  arc A140 (55.3768, 216.4612) -> (58.0942, 213.9503) centre (59.1424, 217.8105) ccw
  circle A141 centre (0, 0) radius 276.5765
  constraint coincident A0.centre A3.centre
extrude "Extrude6" add sketch "Sketch6" along normal blind 40 separate body contours A141 makes body 2
copy_body "CopyPasteBodies1" bodies 1 2 makes body 3 makes body 4
move_body "Move1" bodies 3 4 to x (1, 0, 0) y (0, 1, 0) z (0, 0, 1) at (0, 0, 0)
copy_body "CopyPasteBodies2" bodies 2 1 4 3 makes body 5 makes body 6 makes body 7 makes body 8
move_body "Move2" bodies 5 6 7 8 to x (1, 0, 0) y (0, 1, 0) z (0, 0, 1) at (2000, 0, 0)
sketch "Sketch7" plane through (0, 0, 50) normal (0, 0, 1) x (1, 0, 0)
  circle A0 centre (0, 0) radius 99.7546
  circle A1 centre (0, 0) radius 274.7781
  line L0 (0, -264.8389) -> (2000, -264.8389)
  arc A2 (2000, -264.8389) -> (2000, 264.8389) centre (2000, 0) ccw
  line L1 (2000, 264.8389) -> (0, 264.8389)
  arc A3 (0, 264.8389) -> (0, -264.8389) centre (0, 0) ccw
  line L2 (0, 0) -> (2000, 0) construction
  line L3 (0, -242.279) -> (2000, -242.279)
  arc A4 (2000, -242.279) -> (2000, 242.279) centre (2000, 0) ccw
  line L4 (2000, 242.279) -> (0, 242.279)
  arc A5 (0, 242.279) -> (0, -242.279) centre (0, 0) ccw
  line L5 (0, 0) -> (2000, 0) construction
  constraint tangent L0 A2
  constraint tangent A2 L1
  constraint parallel L0 L1
  constraint tangent L1 A3
  constraint tangent L0 A3
  constraint horizontal L2
  constraint coincident A0.centre A1.centre
  constraint tangent L3 A4
  constraint tangent A4 L4
  constraint parallel L3 L4
  constraint tangent L4 A5
  constraint tangent L3 A5
  constraint coincident A2.centre L2.end
  constraint parallel L2 L5
surface "Extrude7" add extruded along (0, 0, 1) between 0 and -1200 path "Sketch7" along L3 A4 L4 A5 L0 A2 L1 A3 separate body makes body 9 at (666.6667, -242.279, -750) makes body 10 at (666.6667, -264.8389, -750)
